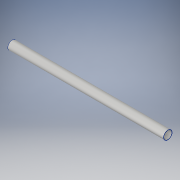
# Autodesk Inventor part: airframe
Saved by Autodesk Inventor 2017 SP1 (Build 210196100, 196)
## iProperties
Created: 2016-10-21
Part Number: airframe
Material: Aluminum 6061
Document SubType Name: Modeling
Designer: cflannery
Density: 2.7 g/cm^3
Appearance: Aluminum - Flat
Author: cflannery
Autodesk Inventor part; units mm, degrees
ref_plane "YZ Plane" through (0, 0, 0) normal (1, 0, 0) x (0, 1, 0)
ref_plane "XZ Plane" through (0, 0, 0) normal (0, 1, 0) x (-1, 0, 0)
ref_plane "XY Plane" through (0, 0, 0) normal (0, 0, 1) x (1, 0, 0)
sketch "Sketch1" plane through (0, 0, 0) normal (0, 0, 1) x (1, 0, 0)
  line L0 (0, 101.6) -> (3657.6, 101.6)
  line L1 (3657.6, 101.6) -> (3657.6, 0)
  line L2 (0, 101.6) -> (0, 0)
  line L3 (0, 0) -> (3657.6, 0)
  dimension "d0" = 101.6
  dimension "d1" = 3657.6
  constraints: 8 end point, 2 horizontal, 1 horizontal alignment, 1 perpendicular, 1 vertical
  measures "d0" distance of L0.start L2.end
  measures "d1" distance of L0.start L0.end
revolve "Revolution1" add sketch "Sketch1" angle 360 about axis through (0, 0, 0) along (1, 0, 0)
shell "Shell1" thickness 6.35 removed faces 2 at (0, -18.1407, 15.8994) at (3657.6, -41.6356, 16.7199)
body "Solid1"
